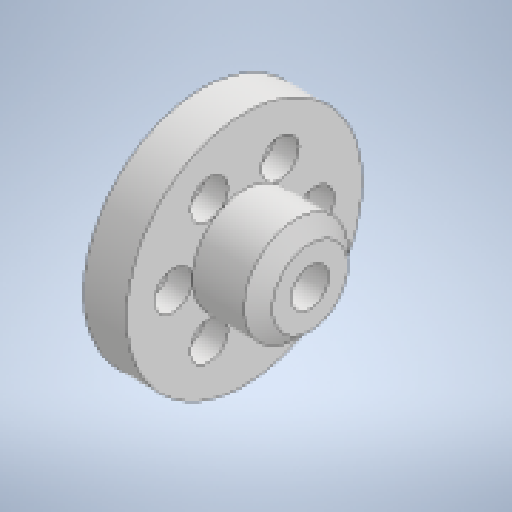
# Autodesk Inventor part: 导轮架
Saved by Autodesk Inventor 2025.1 (Build 291241000, 241)
## iProperties
Created: 2025-08-27
Part Number: 导轮架
Material: 常规
Document SubType Name: Modeling
Designer: Piw
Density: 1 g/cm^3
Appearance: 默认
Author: Piw
Autodesk Inventor part; units mm, degrees
ref_plane "YZ Plane" through (0, 0, 0) normal (1, 0, 0) x (0, 1, 0)
ref_plane "XZ Plane" through (0, 0, 0) normal (0, 1, 0) x (-1, 0, 0)
ref_plane "XY Plane" through (0, 0, 0) normal (0, 0, 1) x (1, 0, 0)
sketch "草图1" plane through (0, 0, 0) normal (1, 0, 0) x (0, 1, 0)
  circle A0 centre (0, 0) radius 25
  circle A1 centre (0, 0) radius 7.5
  circle A2 centre (0, 0) radius 15 construction
  circle A3 centre (0, -15) radius 2.1
  line L0 (0, 0) -> (0, -7.5) construction
  circle A4 centre (12.9904, -7.5) radius 2.1
  circle A5 centre (12.9904, 7.5) radius 2.1
  circle A6 centre (0, 15) radius 2.1
  circle A7 centre (-12.9904, 7.5) radius 2.1
  circle A8 centre (-12.9904, -7.5) radius 2.1
  dimension "d1" = 15
  dimension "d4" = 30
  dimension "d0" = 50
  dimension "d5" = 4.2
  dimension "d8" = 360
  constraints: 7 centre point, 3 coincident, 2 end point, 2 vertical alignment, 1 point on line, 1 vertical, 17 other
  measures "d0" diameter of A0
  measures "d5" diameter of A3
extrude "拉伸1" add sketch "草图1" along normal blind 6
sketch "草图2" plane through (6, 0, 0) normal (1, 0, 0) x (0, 0, -1)
  circle A0 centre (0, 0) radius 25 projected
  circle A1 centre (7.5, 12.9904) radius 2.1 projected
  circle A2 centre (15, 0) radius 2.1 projected
  circle A3 centre (7.5, -12.9904) radius 2.1 projected
  circle A4 centre (-7.5, -12.9904) radius 2.1 projected
  circle A5 centre (0, 0) radius 7.5 projected
  circle A6 centre (-15, 0) radius 2.1 projected
  circle A7 centre (-7.5, 12.9904) radius 2.1 projected
  circle A8 centre (15, 0) radius 4
  circle A9 centre (7.5, 12.9904) radius 4
  circle A10 centre (-7.5, 12.9904) radius 4
  circle A11 centre (-15, 0) radius 4
  circle A12 centre (-7.5, -12.9904) radius 4
  circle A13 centre (7.5, -12.9904) radius 4
  dimension "d10" = 8
  dimension "d13" = 360
  constraints: 6 centre point, 1 coincident, 13 other
  measures "d10" diameter of A8
extrude "拉伸2" add sketch "草图2" along normal blind 5 contours A0
sketch "草图3" plane through (11, 0, 0) normal (1, 0, 0) x (0, 0, -1)
  circle A0 centre (0, 0) radius 4
  circle A1 centre (0, 0) radius 25 projected
  circle A2 centre (7.5, -12.9904) radius 4 projected
  circle A3 centre (15, 0) radius 4 projected
  circle A4 centre (7.5, 12.9904) radius 4 projected
  circle A5 centre (-7.5, 12.9904) radius 4 projected
  circle A6 centre (-15, 0) radius 4 projected
  circle A7 centre (-7.5, -12.9904) radius 4 projected
  circle A8 centre (0, 0) radius 11
  dimension "d17" = 8
  constraints: 2 centre point, 2 coincident, 1 tangent
  measures "d17" diameter of A0
extrude "拉伸3" add sketch "草图3" along normal blind 12.9 contours A8
chamfer "倒角1" distance 2 angle 45 1 edges at (23.9, 0, 11)
chamfer "倒角2" distance 2 angle 45 1 edges at (11, 0, 25)
sketch "草图4" plane through (11, 0, 0) normal (1, 0, 0) x (0, 0, -1)
  circle A0 centre (-15, 0) radius 4 projected
  arc A1 (-5.5, 9.5263) -> (-11, 0) centre (0, 0) ccw projected
  circle A2 centre (-7.5, 12.9904) radius 4 projected
  arc A3 (5.5, 9.5263) -> (-5.5, 9.5263) centre (0, 0) ccw projected
  circle A4 centre (7.5, 12.9904) radius 4 projected
  arc A5 (11, 0) -> (5.5, 9.5263) centre (0, 0) ccw projected
  circle A6 centre (15, 0) radius 4 projected
  arc A7 (5.5, -9.5263) -> (11, 0) centre (0, 0) ccw projected
  circle A8 centre (7.5, -12.9904) radius 4 projected
  arc A9 (-5.5, -9.5263) -> (5.5, -9.5263) centre (0, 0) ccw projected
  circle A10 centre (-7.5, -12.9904) radius 4 projected
  arc A11 (-11, 0) -> (-5.5, -9.5263) centre (0, 0) ccw projected
  circle A12 centre (0, 0) radius 23 projected
  constraints: 2 horizontal alignment, 4 other
extrude "拉伸4" add sketch "草图4" along normal blind 1
chamfer "倒角3" distance 1 angle 45 1 edges at (12, 0, 23)
